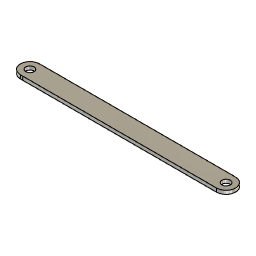
ハンドル (Autodesk Fusion 360 design; units mm, degrees)
Autodesk Fusion 360 part; units mm, degrees
note: some values were not read from the file. Set by a fixed rule: which sketch regions a step uses.
sketch "スケッチ1" plane through (0, 0, 0) normal (0, 0, 1) x (1, 0, 0)
  line L0 (0, 0) -> (82.327, 0)
  circle A0 centre (0, 0) radius 1.75
  circle A1 centre (82.327, 0) radius 1.75
  circle A2 centre (0, 0) radius 4
  circle A3 centre (82.327, 0) radius 4
  line L1 (5, 4) -> (0, 4)
  line L2 (5, 4) -> (82.327, 4)
  line L3 (1, -4) -> (0, -4)
  line L4 (1, -4) -> (82.327, -4)
  dimension "d1" = 82.327
  dimension "d2" = 3.5
  dimension "d3" = 3.5
  dimension "d4" = 8
  dimension "d5" = 8
  constraint coincident L0.start A0.centre
  constraint horizontal L0
  constraint coincident L0.end A1.centre
  constraint concentric A1 A3
  constraint coincident A2 L1.end
  constraint tangent A2 L1
  constraint coincident A3 L2.end
  constraint tangent A3 L2
  constraint coincident A2 L3.end
  constraint tangent A2 L3
  constraint coincident A3 L4.end
  constraint tangent A3 L4
  measures "d1" distance of L0.start L0.end
  measures "d2" diameter of A0
  measures "d3" diameter of A1
  measures "d4" diameter of A2
  measures "d5" diameter of A3
extrude "押し出し1" add sketch "スケッチ1" along normal blind 2
extrude "押し出し2" cut 1 faces at (28.9168, -0.2531, 2) along direction (0, 0, -1) blind 0.5
